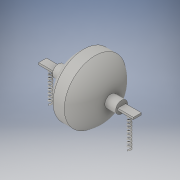
# Autodesk Inventor part: WireCounterPiece1
Saved by Autodesk Inventor 2016 (Build 200138000, 138)
## iProperties
Created: 2015-12-01
Part Number: WireCounterPiece1
Material: Generic
Document SubType Name: Modeling
Designer: Javier
Density: 1 g/cm^3
Appearance: Default
Author: Javier
Autodesk Inventor part; units mm, degrees
sketch "Sketch2" plane through (0, 0, 0) normal (0, 0, 1) x (1, 0, 0)
  line L0 (-4.9529, -9.9058) -> (-4.9529, 14.8588)
  line L1 (-4.9529, 14.8588) -> (4.098, 14.8588)
  line L2 (4.098, 14.8588) -> (4.098, -9.9058)
  line L3 (4.098, -9.9058) -> (-4.9529, -9.9058)
  line L4 (-17.6529, -9.9058) -> (-4.9529, -9.9058)
  line L5 (4.098, -9.9058) -> (16.798, -9.9058)
  arc A0 (-4.9529, 14.8588) -> (-17.6529, -9.9058) centre (14.807, -10.9134) ccw
  arc A1 (16.798, -9.9058) -> (4.098, 14.8588) centre (-10.0274, -8.0239) ccw
  point P0 (0, 0)
  dimension "d6" = 12.7
  dimension "d7" = 24.7646
  dimension "d9" = 12.7
  dimension "d10" = 24.7646
  constraints: 12 end point, 4 point on circle, 2 centre point, 2 perpendicular, 1 horizontal, 1 parallel
  measures "d6" distance of L4.start L0.start
  measures "d7" vertical distance of L4.start L0.end
  measures "d9" distance of L2.end L5.end
  measures "d10" vertical distance of L5.end L1.end
revolve "Revolution1" add sketch "Sketch2" angle 360 about axis through (4.098, -9.9058, 0) along (-1, 0, 0)
sketch "Sketch3" plane through (0, 0, 0) normal (1, 0, 0) x (0, 1, 0)
  line L0 (19.05, 0) -> (-39.6875, 0)
  line L1 (-10.3188, -28.575) -> (-10.3188, 39.0535)
  circle A0 centre (-10.3188, 0) radius 4.7625
  point P0 (0, 0)
  constraints: 4 end point, 1 centre point, 1 horizontal, 1 midpoint, 1 point on line, 1 vertical
extrude "Extrusion2" add sketch "Sketch3" along normal mid plane 50.8
ref_plane "Work Plane2" through (25.4, 0, 0) normal (1, 0, 0) x (0, 1, 0)
sketch "Sketch4" plane through (25.4, 0, 0) normal (1, 0, 0) x (0, 1, 0)
  line L0 (-11.1125, 3.175) -> (-9.525, 3.175)
  line L1 (-9.525, 3.175) -> (-9.525, -3.175)
  line L2 (-9.525, -3.175) -> (-11.1125, -3.175)
  line L3 (-11.1125, -3.175) -> (-11.1125, 3.175)
  point P0 (0, 0)
  constraints: 8 end point, 2 parallel, 1 horizontal, 1 perpendicular
extrude "Extrusion3" add sketch "Sketch4" along normal blind 12.7
ref_plane "Work Plane3" through (-25.4, 0, 0) normal (1, 0, 0) x (0, 1, 0)
sketch "Sketch5" plane through (-25.4, 0, 0) normal (1, 0, 0) x (0, 1, 0)
  line L0 (-11.1125, 3.175) -> (-11.1125, -3.175) projected
  line L1 (-9.525, 3.175) -> (-11.1125, 3.175) projected
  line L2 (-11.1125, -3.175) -> (-9.525, -3.175)
  line L3 (-9.525, -3.175) -> (-9.525, 3.175)
  line L4 (-9.525, 3.175) -> (-11.1125, 3.175)
  line L5 (-11.1125, 3.175) -> (-11.1125, -3.175)
  point P0 (0, 0)
  constraints: 8 end point, 2 parallel, 1 horizontal, 1 perpendicular
extrude "Extrusion4" add sketch "Sketch5" against normal blind 12.7
ref_plane "Work Plane4" through (-31.75, 0, 0) normal (1, 0, 0) x (0, 1, 0)
sketch "Sketch6" plane through (-31.75, 0, 0) normal (1, 0, 0) x (0, 1, 0)
  line L0 (-11.1125, -3.175) -> (-11.1125, 3.175) projected
  line L1 (-11.1125, 0) -> (-36.5125, 0)
  line L2 (-36.5125, 0) -> (-36.5125, 1.1226)
  circle A0 centre (-36.5125, 1.1226) radius 0.635
  point P0 (0, 0)
  dimension "d23" = 1.27
  dimension "d24" = 25.4
  constraints: 4 end point, 1 centre point, 1 coincident, 1 horizontal, 1 midpoint, 1 vertical
  measures "d23" diameter of A0
  measures "d24" distance of L1.start L1.end
coil "Coil1" sketch "Sketch6" operation add axis through (-31.75, -11.1125, 0) along (0, 1, 0) pitch 2.54 turns 10 hand right
ref_plane "Work Plane5" through (31.75, 0, 0) normal (1, 0, 0) x (0, 1, 0)
sketch "Sketch7" plane through (31.75, 0, 0) normal (1, 0, 0) x (0, 1, 0)
  line L0 (-11.1125, 3.175) -> (-11.1125, -3.175) projected
  line L1 (-11.1125, 0) -> (-36.5125, 0)
  circle A0 centre (-36.5125, 1.1226) radius 0.635 projected
  line L2 (-36.5125, 0) -> (-36.5125, 1.1226)
  circle A1 centre (-36.5125, 1.1226) radius 0.635
  point P0 (0, 0)
  point P1 (-35.8775, 1.1226)
  constraints: 4 end point, 1 centre point, 1 coincident, 1 horizontal, 1 horizontal alignment, 1 midpoint, 1 perpendicular, 1 other
coil "Coil2" sketch "Sketch7" operation add axis through (31.75, -11.1125, 0) along (0, 1, 0) pitch 2.54 turns 10 hand right
body "Solid2"
